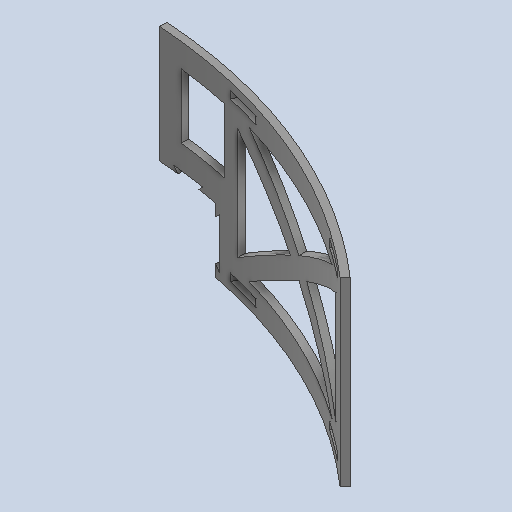
# Autodesk Inventor part: Battery Module Third Iteration Inner Wall
Saved by Autodesk Inventor 2023 (Build 270158000, 158)
## iProperties
Created: 2023-03-05
Part Number: Battery Module Third Iteration Inner Wall
Material: PLA Plastic
Document SubType Name: Modeling
Designer: mihal
Density: 1.25002 g/cm^3
Appearance: Generic
Mass: 21.7749 g
Surface Area: 156.054 cm^2
Volume: 17.4196 cm^3
Author: mihal
Autodesk Inventor part; units mm, degrees
sketch "Sketch1" plane through (0, 0, 0) normal (0, 1, 0) x (-1, 0, 0)
  circle A0 centre (0, 0) radius 215
  circle A1 centre (0, 0) radius 315
  line L0 (0, 0) -> (0, -315)
  line L1 (0, 0) -> (-222.7386, -222.7386)
  line L2 (-141.0509, -162.2641) -> (-211.8794, -233.0926)
  line L3 (-15, -214.4761) -> (-15, -314.6427)
  circle A2 centre (0, 0) radius 219.5
  circle A3 centre (0, 0) radius 310.5
  circle A4 centre (0, 0) radius 222.5
  point P0 (-152.028, -152.028)
  point P1 (0, -215)
  point P2 (0, -312.5)
  point P3 (0, -217.5)
  point P4 (-153.7957, -153.7957)
  point P5 (-220.9709, -220.9709)
  point P6 (-210.1096, -231.3228)
  point P7 (-15, -312.1398)
  point P8 (-15, -216.9821)
  point P9 (-142.8229, -164.0361)
  point P10 (-207.7734, -228.9866)
  point P11 (-15, -308.8359)
  point P12 (-15, -220.2899)
  point P13 (-145.1619, -166.3751)
  point P14 (-144.2405, -165.4537)
  point P15 (-15, -218.9869)
  point P16 (-146.3667, -167.5799)
  point P17 (-15, -221.9938)
  dimension "d0" = 430
  dimension "d1" = 630
  dimension "d2" = 45
  dimension "d3" = 15
  dimension "d4" = 15
  dimension "d5" = 4.5
  dimension "d6" = 4.5
  dimension "d13" = 3
  constraints: 8 end point, 6 point on circle, 5 centre point, 5 coincident, 2 parallel, 1 vertical
  measures "d0" diameter of A0
  measures "d1" diameter of A1
  measures "d2" angle of L1 L0
  measures "d3" distance between parallel lines of L2 L1
  measures "d4" distance between parallel lines of L3 L0
  measures "d5" radial gap between concentric circles of A0 A2
  measures "d6" radial gap between concentric circles of A3 A1
  measures "d13" radial gap between concentric circles of A2 A4
extrude "Extrusion1" add sketch "Sketch1" along normal blind 76 contours A2 L3 A4 L2
sketch "Sketch3" plane through (0, 0, 0) normal (0, 0, 1) x (1, 0, 0)
  line L0 (15, 0) -> (144.2405, 0) projected
  line L1 (144.2405, 0) -> (144.2405, 76) projected
  line L2 (15, 76) -> (144.2405, 76) projected
  line L3 (15, 0) -> (15, 76) projected
  line L4 (15, 0) -> (42, 0)
  line L5 (42, 0) -> (42, 27)
  line L6 (42, 27) -> (15, 27)
  line L7 (15, 27) -> (15, 0)
  line L8 (42, 5) -> (44, 3)
  line L9 (44, 3) -> (44, 24)
  line L10 (44, 24) -> (42, 22)
  line L11 (23.5, 27) -> (21.5, 29)
  line L12 (21.5, 29) -> (35.5, 29)
  line L13 (35.5, 29) -> (33.5, 27)
  point P0 (0, 0)
  dimension "d14" = 27
  dimension "d15" = 27
  dimension "d18" = 2
  dimension "d19" = 2
  dimension "d20" = 2
  dimension "d21" = 3
  dimension "d22" = 21
  dimension "d23" = 2
  dimension "d24" = 2
  dimension "d25" = 2
  dimension "d26" = 6.5
  dimension "d27" = 6.5
  constraints: 20 end point, 4 point on line, 3 parallel, 2 horizontal, 1 perpendicular
  measures "d14" distance of L6.end L5.end
  measures "d15" distance of L5.end L4.end
  measures "d18" distance between parallel lines of L5 L9
  measures "d19" horizontal distance of L9.end L10.end
  measures "d20" horizontal distance of L8.end L8.start
  measures "d21" distance from line of L0 L8.end
  measures "d22" distance of L8.end L9.end
  measures "d23" distance between parallel lines of L6 L12
  measures "d24" horizontal distance of L11.end L11.start
  measures "d25" horizontal distance of L12.end L13.end
  measures "d26" horizontal distance of L6.end L11.end
  measures "d27" horizontal distance of L5.end L12.end
extrude "Extrusion3" cut sketch "Sketch3" against normal up to surface contours L3 L6 L5 L0 | L5 L10 L9 L8 | L11 L12 L13 L6 round surface about axis through (0, 0, 0) along (0, 1, 0) radius 222.5 far side no
sketch "Sketch7" plane through (0, 0, 0) normal (0, 0, 1) x (1, 0, 0)
  line L0 (42, 5) -> (42, 0) projected
  line L1 (42, 0) -> (144.2405, 0) projected
  line L2 (144.2405, 0) -> (144.2405, 76) projected
  line L3 (15, 76) -> (144.2405, 76) projected
  line L4 (15, 27) -> (15, 76) projected
  line L5 (15, 27) -> (23.5, 27) projected
  line L6 (23.5, 27) -> (21.5, 29) projected
  line L7 (21.5, 29) -> (35.5, 29) projected
  line L8 (35.5, 29) -> (33.5, 27) projected
  line L9 (33.5, 27) -> (42, 27) projected
  line L10 (42, 27) -> (42, 22) projected
  line L11 (42, 22) -> (44, 24) projected
  line L12 (44, 24) -> (44, 3) projected
  line L13 (44, 3) -> (42, 5) projected
  line L14 (15, 39) -> (54, 39)
  line L15 (54, 39) -> (54, 0)
  line L16 (25, 39) -> (25, 66)
  line L17 (25, 66) -> (134.2405, 66)
  line L18 (134.2405, 66) -> (134.2405, 10)
  line L19 (134.2405, 10) -> (54, 10)
  line L20 (54, 39) -> (54, 66)
  line L21 (54, 14.573) -> (127.6881, 66)
  line L22 (60.5524, 10) -> (134.2405, 61.427)
  line L23 (54, 10) -> (134.2405, 66) construction
  line L24 (54, 66) -> (134.2405, 10) construction
  line L25 (54, 61.427) -> (127.6881, 10)
  line L26 (60.5524, 66) -> (134.2405, 14.573)
  line L27 (46.5, 66) -> (46.5, 39)
  point P0 (0, 0)
  point P1 (54, 52.5)
  point P2 (94.1203, 42.573)
  point P3 (100.6727, 38)
  point P4 (87.5678, 38)
  point P5 (94.1203, 33.427)
  point P6 (46.5, 52.5)
  dimension "d100" = 10
  dimension "d101" = 10
  dimension "d102" = 10
  dimension "d103" = 10
  dimension "d104" = 10
  dimension "d105" = 10
  dimension "d113" = 7.5
  dimension "d114" = 7.5
  dimension "d115" = 7.5
  constraints: 28 end point, 15 point on line, 5 perpendicular, 4 parallel, 2 horizontal, 2 midpoint, 1 vertical, 2 other
  measures "d100" distance between parallel lines of L12 L15
  measures "d101" distance between parallel lines of L1 L19
  measures "d102" distance between parallel lines of L2 L18
  measures "d103" distance between parallel lines of L3 L17
  measures "d104" distance between parallel lines of L4 L16
  measures "d105" distance between parallel lines of L7 L14
  measures "d113" distance from line of L20 point (46.5, 52.5)
  measures "d114" distance between parallel lines of L22 L21
  measures "d115" distance between parallel lines of L25 L26
extrude "Extrusion7" cut sketch "Sketch7" against normal up to surface contours L15 L20 L25 L21 | L22 L25 L19 | L14 L16 L17 L27 | L26 L17 L21 | L22 L18 L26 round surface about axis through (0, 0, 0) along (0, 1, 0) radius 222.5 far side no
ref_plane "Work Plane4" through (0, 71, 0) normal (0, 1, 0) x (1, 0, 0)
ref_plane "Work Plane6" through (21.8883, 0, -238.6236) normal (0.3826834, 0, -0.9238795) x (0, 1, 0)
ref_plane "Work Plane5" through (15, 0, -221.9938) normal (0.3826834, 0, -0.9238795) x (0, 1, 0)
ref_plane "Work Plane7" through (144.2405, 0, -165.4537) normal (-0.3826834, 0, 0.9238795) x (0, 1, 0)
sketch "Sketch10" plane through (144.2405, 0, -165.4537) normal (-0.3826834, 0, 0.9238795) x (0, 1, 0)
  ellipse E0 centre (-32.2597, 69.9445) end of major axis (115.4894, -147.8322) minor radius 48.896 (33.427, 58.8736) -> (10, 94.7408) ccw projected
  ellipse E1 centre (99.1138, 69.9445) end of major axis (-48.6353, -147.8322) minor radius 48.896 (33.427, 58.8736) -> (10, 20.2998) ccw projected
  line L0 (10, 20.2998) -> (10, 94.7408) projected
  line L1 (14.573, 101.4724) -> (61.427, 101.4724) projected
  ellipse E2 centre (99.1138, 69.9445) end of major axis (-48.6353, -147.8322) minor radius 48.896 (61.427, 101.4724) -> (38, 66.0674) ccw projected
  ellipse E3 centre (-23.1138, 69.9445) end of major axis (124.6353, -147.8322) minor radius 48.896 (38, 66.0674) -> (14.573, 101.4724) ccw projected
  ellipse E4 centre (108.2597, 69.9445) end of major axis (-39.4894, -147.8322) minor radius 48.896 (66, 94.7408) -> (42.573, 58.8736) ccw projected
  line L2 (66, 94.7408) -> (66, 20.2998) projected
  ellipse E5 centre (-23.1138, 69.9445) end of major axis (124.6353, -147.8322) minor radius 48.896 (66, 20.2998) -> (42.573, 58.8736) ccw projected
  line L3 (66, 109.0766) -> (39, 109.0766) projected
  line L4 (39, 109.0766) -> (39, 130.2999) projected
  line L5 (39, 130.2999) -> (66, 130.2999) projected
  line L6 (66, 130.2999) -> (66, 109.0766) projected
  ellipse E6 centre (108.2597, 69.9445) end of major axis (-39.4894, -147.8322) minor radius 48.896 (38, 51.5782) -> (14.573, 12.3813) ccw projected
  ellipse E7 centre (-32.2597, 69.9445) end of major axis (115.4894, -147.8322) minor radius 48.896 (61.427, 12.3813) -> (38, 51.5782) ccw projected
  line L7 (61.427, 12.3813) -> (14.573, 12.3813) projected
  line L8 (5, 113.5885) -> (0, 113.5885) projected
  line L9 (0, 113.5885) -> (0, 0) projected
  line L10 (0, 0) -> (76, 0) projected
  line L11 (76, 139.8889) -> (76, 0) projected
  line L12 (27, 139.8889) -> (76, 139.8889) projected
  line L13 (27, 139.8889) -> (27, 131.7495) projected
  ellipse E8 centre (50.5, 69.9445) end of major axis (-164.7824, -145.3379) minor radius 60.5599 (29, 133.6761) -> (27, 131.7495) ccw projected
  line L14 (29, 133.6761) -> (29, 120.0399) projected
  ellipse E9 centre (-6.5, 69.9445) end of major axis (208.7824, -145.3379) minor radius 60.5599 (29, 120.0399) -> (27, 122.0095) ccw projected
  line L15 (27, 122.0095) -> (27, 113.5885) projected
  line L16 (27, 113.5885) -> (22, 113.5885) projected
  ellipse E10 centre (-20, 69.9445) end of major axis (195.2824, -145.3379) minor radius 60.5599 (24, 111.5878) -> (22, 113.5885) ccw projected
  line L17 (24, 111.5878) -> (3, 111.5878) projected
  ellipse E11 centre (47, 69.9445) end of major axis (-168.2824, -145.3379) minor radius 60.5599 (5, 113.5885) -> (3, 111.5878) ccw projected
  line L18 (61.427, 101.4724) -> (76, 101.4724) construction
  line L19 (61.427, 12.3813) -> (76, 12.3813) construction
  line L20 (72.8, 139.8889) -> (72.8, 0) construction
  line L21 (66, 20.2998) -> (72.8, 20.2998) construction
  line L22 (69.4, 20.2998) -> (69.4, 12.3813) construction
  line L23 (69.4, 16.3406) -> (59.151, 16.3406) construction
  line L24 (69.4, 16.3406) -> (72.8, 16.3406) construction
  line L25 (69.6, 23.9406) -> (72.8, 23.9406)
  line L26 (72.8, 23.9406) -> (72.8, 8.7406)
  line L27 (72.8, 8.7406) -> (69.6, 8.7406)
  line L28 (69.6, 8.7406) -> (69.6, 23.9406)
  line L29 (69.6, 23.9406) -> (72.8, 8.7406) construction
  line L30 (72.8, 23.9406) -> (69.6, 8.7406) construction
  line L31 (66, 94.7408) -> (72.8, 94.7408) construction
  line L32 (69.4, 94.7408) -> (69.4, 101.4724) construction
  line L33 (69.4, 98.1066) -> (59.1335, 98.1066) construction
  line L34 (69.4, 98.1066) -> (72.8, 98.1066) construction
  line L35 (3.2, 0) -> (3.2, 113.5885) construction
  line L36 (14.573, 101.4724) -> (0, 101.4724) construction
  line L37 (10, 94.7408) -> (0, 94.7408) construction
  line L38 (5, 94.7408) -> (5, 101.4724) construction
  line L39 (5, 98.1066) -> (16.8665, 98.1066) construction
  line L40 (5, 98.1066) -> (0, 98.1066) construction
  line L41 (10, 20.2998) -> (0, 20.2998) construction
  line L42 (14.573, 12.3813) -> (0, 12.3813) construction
  line L43 (5, 20.2998) -> (5, 12.3813) construction
  line L44 (5, 16.3406) -> (16.849, 16.3406) construction
  line L45 (5, 16.3406) -> (0, 16.3406) construction
  line L46 (72.8, 105.7066) -> (69.6, 105.7066)
  line L47 (69.6, 105.7066) -> (69.6, 90.5066)
  line L48 (69.6, 90.5066) -> (72.8, 90.5066)
  line L49 (72.8, 90.5066) -> (72.8, 105.7066)
  line L50 (72.8, 105.7066) -> (69.6, 90.5066) construction
  line L51 (69.6, 105.7066) -> (72.8, 90.5066) construction
  line L52 (3.2, 105.7066) -> (6.4, 105.7066)
  line L53 (6.4, 105.7066) -> (6.4, 90.5066)
  line L54 (6.4, 90.5066) -> (3.2, 90.5066)
  line L55 (3.2, 90.5066) -> (3.2, 105.7066)
  line L56 (3.2, 105.7066) -> (6.4, 90.5066) construction
  line L57 (6.4, 105.7066) -> (3.2, 90.5066) construction
  line L58 (6.4, 23.9406) -> (3.2, 23.9406)
  line L59 (3.2, 23.9406) -> (3.2, 8.7406)
  line L60 (3.2, 8.7406) -> (6.4, 8.7406)
  line L61 (6.4, 8.7406) -> (6.4, 23.9406)
  line L62 (6.4, 23.9406) -> (3.2, 8.7406) construction
  line L63 (3.2, 23.9406) -> (6.4, 8.7406) construction
  point P0 (0, 69.9445)
  point P1 (71.2, 16.3406)
  point P2 (71.2, 98.1066)
  point P3 (4.8, 98.1066)
  point P4 (4.8, 16.3406)
  point P5 (3.2, 16.3406)
  point P6 (3.2, 98.1066)
  dimension "d128" = 3.2
  dimension "d131" = 3.2
  dimension "d132" = 15.2
  dimension "d133" = 3.2
  dimension "d134" = 3.2
  dimension "d135" = 15.2
  dimension "d136" = 3.2
  dimension "d137" = 15.2
  dimension "d138" = 3.2
  dimension "d139" = 15.2
  constraints: 92 end point, 33 point on line, 20 midpoint, 18 perpendicular, 10 parallel, 5 horizontal, 2 coincident, 16 other
  measures "d128" distance between parallel lines of L11 L20
  measures "d131" distance of L26.end L27.end
  measures "d132" distance of L25.end L26.end
  measures "d133" distance between parallel lines of L9 L35
  measures "d134" distance of L48.end L47.end
  measures "d135" distance of L47.end L46.end
  measures "d136" distance of L53.end L54.end
  measures "d137" distance of L52.end L53.end
  measures "d138" distance of L60.end L59.end
  measures "d139" distance of L59.end L58.end
extrude "Extrusion9" cut sketch "Sketch10" against normal up to surface contours L25 L26 L27 L28 | L49 L48 L47 L46 | L52 L53 L54 L55 | L61 L60 L59 L58 round surface about axis through (0, 0, 0) along (0, 1, 0) radius 222.5 far side no
equation "\"d134\" = d131"
equation "\"d135\" = d132"
equation "\"d136\" = d131"
equation "\"d137\" = d132"
equation "\"d138\" = d131"
equation "\"d139\" = d132"
body "Solid1"
